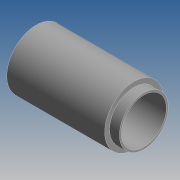
# Autodesk Inventor part: P008_CanonBout
Saved by Autodesk Inventor 2020 (Build 240168000, 168)
## iProperties
Created: 2021-10-15
Part Number: P008_CanonBout
Material: Générique
Document SubType Name: Modeling
Designer: gabri
Density: 1 g/cm^3
Appearance: Par défaut
Author: gabri
Autodesk Inventor part; units mm, degrees
ref_plane "YZ Plane" through (0, 0, 0) normal (1, 0, 0) x (0, 1, 0)
ref_plane "XZ Plane" through (0, 0, 0) normal (0, 1, 0) x (-1, 0, 0)
ref_plane "XY Plane" through (0, 0, 0) normal (0, 0, 1) x (1, 0, 0)
sketch "Esquisse9" plane through (0, 0, 0) normal (0, 1, 0) x (-1, 0, 0)
  line L0 (0, 0) -> (100, 0)
  line L1 (120, 0) -> (-20, 0) construction
  dimension "d20" = 100
  constraints: 2 end point, 1 horizontal
  measures "d20" distance of L0.start L0.end
sketch "Esquisse10" plane through (0, 0, 0) normal (1, 0, 0) x (0, 1, 0)
  circle A0 centre (0, 0) radius 30
  circle A1 centre (0, 0) radius 23
  dimension "d22" = 60
  dimension "d23" = 46
  constraints: 2 centre point, 2 coincident
  measures "d22" diameter of A0
  measures "d23" diameter of A1
sweep "Balayage2" add profiles "Esquisse10" path "Esquisse9"
sketch "Esquisse11" plane through (0, 0, 0) normal (1, 0, 0) x (0, 0, -1)
  circle A0 centre (0, 0) radius 23 construction
  circle A1 centre (0, 0) radius 30 construction
  circle A2 centre (0, 0) radius 23
  circle A3 centre (0, 0) radius 25
  dimension "d26" = 50
  constraints: 2 centre point, 2 coincident, 1 concentric
  measures "d26" diameter of A3
extrude "Extrusion4" add sketch "Esquisse11" along normal blind 10
sketch "Esquisse15" plane through (-100, 0, 0) normal (-1, 0, 0) x (0, 0, 1)
  circle A0 centre (0, 0) radius 23
  circle A1 centre (0, 0) radius 25
  dimension "d41" = 46
  dimension "d42" = 50
  constraints: 2 centre point, 2 coincident
  measures "d41" diameter of A0
  measures "d42" diameter of A1
extrude "Extrusion6" cut sketch "Esquisse15" against normal blind 10
